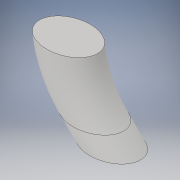
# Autodesk Inventor part: horn
Saved by Autodesk Inventor 2019.3 (Build 233278000, 278)
## iProperties
Created: 2019-02-15
Part Number: horn
Material: Generic
Document SubType Name: Modeling
Designer: Frienddo
Density: 1 g/cm^3
Appearance: Default
Author: Frienddo
Autodesk Inventor part; units mm, degrees
ref_plane "YZ Plane" through (0, 0, 0) normal (1, 0, 0) x (0, 1, 0)
ref_plane "XZ Plane" through (0, 0, 0) normal (0, 1, 0) x (-1, 0, 0)
ref_plane "XY Plane" through (0, 0, 0) normal (0, 0, 1) x (1, 0, 0)
sketch "Sketch1" plane through (0, 0, 0) normal (0, 1, 0) x (-1, 0, 0)
  ellipse E0 centre (0, 0) end of major axis (8.6139, 0) minor radius 6.4109
  constraints: 1 coincident, 2 other
sketch "Sketch2" plane through (0, 0, 0) normal (0, 0, 1) x (1, 0, 0)
  line L0 (0, 0) -> (-4.9939, 4.9402)
  arc A0 (-12.7662, 20.9799) -> (-4.9939, 4.9402) centre (13.8223, 23.9609) ccw
  constraints: 2 end point, 2 point on circle, 1 centre point, 1 tangent
sweep "Sweep1" add profiles "Sketch1" path "Sketch2" keep normal constant yes
body "Solid1"
